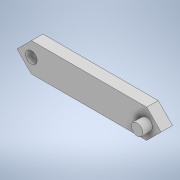
# Autodesk Inventor part: Eslabon_2_inventor
Saved by Autodesk Inventor 2021 (Build 250183000, 183)
## iProperties
Created: 2021-08-13
Part Number: Eslabon_2_inventor
Material: Genérico
Document SubType Name: Modeling
Designer: uriel
Density: 1 g/cm^3
Appearance: Valor por defecto
Author: uriel
Autodesk Inventor part; units mm, degrees
ref_plane "YZ Plane" through (0, 0, 0) normal (1, 0, 0) x (0, 1, 0)
ref_plane "XZ Plane" through (0, 0, 0) normal (0, 1, 0) x (-1, 0, 0)
ref_plane "XY Plane" through (0, 0, 0) normal (0, 0, 1) x (1, 0, 0)
sketch "Boceto1" plane through (0, 0, 0) normal (0, 0, 1) x (1, 0, 0)
  circle A0 centre (0, 0) radius 6
  line L0 (0, 0) -> (0, 15)
  line L1 (0, 15) -> (120, 15)
  line L2 (120, 15) -> (120, -15)
  line L3 (120, -15) -> (0, -15)
  line L4 (0, -15) -> (0, 0)
  circle A1 centre (120, 0) radius 6
  line L5 (120, 0) -> (135, 0)
  line L6 (120, -15) -> (135, 0)
  line L7 (135, 0) -> (120, 15)
  line L8 (0, 0) -> (-15, 0)
  line L9 (-15, 0) -> (0, -15)
  line L10 (-15, 0) -> (0, 15)
  dimension "d0" = 12
  dimension "d1" = 15
  dimension "d2" = 120
  dimension "d3" = 30
  dimension "d4" = 12
  dimension "d5" = 15
  dimension "d6" = 15
  constraints: 22 end point, 4 perpendicular, 2 centre point, 2 horizontal, 1 coincident, 1 midpoint, 1 vertical
  measures "d0" diameter of A0
  measures "d1" distance of L0.start L0.end
  measures "d2" distance of L0.end L1.end
  measures "d3" distance of L1.end L2.end
  measures "d4" diameter of A1
  measures "d5" distance of L5.start L5.end
  measures "d6" distance of L0.start L8.end
extrude "Extrusión1" add sketch "Boceto1" along normal blind 12 contours A0 L0 L1 L2 A1 L3 L4 | A0 L8 L10 L0 | L4 L9 L8 A0 | L7 L5 A1 L2 | L2 A1 L5 L6 | A1 L5 L2 | L2 A1 | L2 L5 A1
sketch "Boceto2" plane through (0, 0, 12) normal (0, 0, 1) x (1, 0, 0)
  line L0 (0, 0) -> (120, 0)
  circle A0 centre (120, 0) radius 6
  dimension "d9" = 120
  dimension "d10" = 12
  constraints: 2 end point, 1 centre point, 1 coincident, 1 horizontal
  measures "d9" distance of L0.start L0.end
  measures "d10" diameter of A0
extrude "Extrusión2" add sketch "Boceto2" along normal blind 10
equation "\"d7\" = d4"
